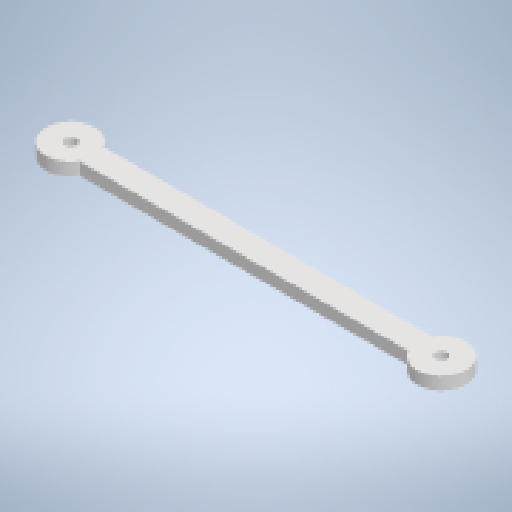
# Autodesk Inventor part: Рычаг головы
Saved by Autodesk Inventor 2023.2 (Build 272271030, 271C)
## iProperties
Created: 2024-02-20
Part Number: Рычаг головы
Material: Типовые
Document SubType Name: Modeling
Designer: I9232
Density: 1 g/cm^3
Appearance: По умолчанию
Author: I9232
Autodesk Inventor part; units mm, degrees
ref_plane "YZ Plane" through (0, 0, 0) normal (1, 0, 0) x (0, 1, 0)
ref_plane "XZ Plane" through (0, 0, 0) normal (0, 1, 0) x (-1, 0, 0)
ref_plane "XY Plane" through (0, 0, 0) normal (0, 0, 1) x (1, 0, 0)
sketch "Эскиз1" plane through (0, 0, 0) normal (0, 1, 0) x (-1, 0, 0)
  arc A0 (39.8038, -3) -> (39.8038, 3) centre (45, 0) ccw
  line L0 (29.2568, 0) -> (27.2769, 0)
  circle A1 centre (45, 0) radius 1.45
  line L1 (0, -3) -> (39.8038, -3)
  line L2 (0, 3) -> (39.8038, 3)
  line L3 (0, -9.1238) -> (0, 12.1062) construction
  arc A2 (-39.8038, 3) -> (-39.8038, -3) centre (-45, 0) ccw
  circle A3 centre (-45, 0) radius 1.45
  line L4 (0, -3) -> (-39.8038, -3)
  line L5 (0, 3) -> (-39.8038, 3)
  point P0 (0, 0)
  dimension "d2" = 2.9
  dimension "d5" = 6
  dimension "d7" = 6
  dimension "d8" = 45
  constraints: 12 end point, 7 symmetric about line, 4 centre point, 4 point on circle, 3 horizontal, 3 point on line, 2 coincident, 1 vertical, 2 other
  measures "d2" diameter of A1
  measures "d5" radius of A0
  measures "d7" distance between parallel lines of L2 L1
  measures "d8" distance of point (0, 0) A0.centre
extrude "Выдавливание1" add sketch "Эскиз1" along normal mid plane 3
fillet "Сопряжение1" radius 10 4 edges at (-39.8038, 0, -3) (-39.8038, 0, 3) (39.8038, 0, 3) (39.8038, 0, -3)
